Autodesk Fusion 360 part; units mm, degrees
(part 7 of 11)
  spline S10 degree 5 poles (-13.755, -25.3425) (-13.7559, -25.3451) (-13.7577, -25.3503) (-13.7602, -25.3581) (-13.7631, -25.3687) (-13.7662, -25.3821) (-13.769, -25.3956) (-13.7716, -25.4092) (-13.774, -25.4229) (-13.7763, -25.4365) (-13.7786, -25.4502) (-13.7807, -25.464) (-13.7827, -25.4778) (-13.7845, -25.4916) (-13.7861, -25.5055) (-13.7876, -25.5194) (-13.7889, -25.5334) (-13.7901, -25.5475) (-13.7912, -25.5615) (-13.7921, -25.5756) (-13.793, -25.5897) (-13.7938, -25.6039) (-13.7945, -25.618) (-13.795, -25.6322) (-13.7955, -25.6465) (-13.7958, -25.6607) (-13.796, -25.675) (-13.7962, -25.6894) (-13.7962, -25.7037) (-13.7961, -25.7181) (-13.796, -25.7325) (-13.7957, -25.7469) (-13.7954, -25.7613) (-13.7949, -25.7758) (-13.7944, -25.7903) (-13.7938, -25.8048) (-13.7931, -25.8193) (-13.7923, -25.8339) (-13.7914, -25.8484) (-13.7905, -25.863) (-13.7894, -25.8776) (-13.7883, -25.8923) (-13.7871, -25.9069) (-13.7857, -25.9216) (-13.7844, -25.9362) (-13.7829, -25.9509) (-13.7813, -25.9656) (-13.7797, -25.9804) (-13.778, -25.9951) (-13.7762, -26.0099) (-13.7743, -26.0247) (-13.7724, -26.0394) (-13.7704, -26.0542) (-13.7683, -26.0691) (-13.7661, -26.0839) (-13.7638, -26.0987) (-13.7615, -26.1136) (-13.7591, -26.1285) (-13.7566, -26.1433) (-13.754, -26.1582) (-13.7514, -26.1731) (-13.7487, -26.1881) (-13.7459, -26.203) (-13.743, -26.2179) (-13.7401, -26.2329) (-13.7371, -26.2478) (-13.734, -26.2628) (-13.7309, -26.2778) (-13.7277, -26.2928) (-13.7244, -26.3078) (-13.721, -26.3228) (-13.7183, -26.3348) (-13.7162, -26.3438) (-13.7148, -26.3498) (-13.714, -26.3528) knots 0 0 0 0 0 0 0.01428571 0.02857143 0.04285714 0.05714286 0.07142857 0.08571429 0.1 0.11428571 0.12857143 0.14285714 0.15714286 0.17142857 0.18571429 0.2 0.21428571 0.22857143 0.24285714 0.25714286 0.27142857 0.28571429 0.3 0.31428571 0.32857143 0.34285714 0.35714286 0.37142857 0.38571429 0.4 0.41428571 0.42857143 0.44285714 0.45714286 0.47142857 0.48571429 0.5 0.51428571 0.52857143 0.54285714 0.55714286 0.57142857 0.58571429 0.6 0.61428571 0.62857143 0.64285714 0.65714286 0.67142857 0.68571429 0.7 0.71428571 0.72857143 0.74285714 0.75714286 0.77142857 0.78571429 0.8 0.81428571 0.82857143 0.84285714 0.85714286 0.87142857 0.88571429 0.9 0.91428571 0.92857143 0.94285714 0.95714286 0.97142857 0.98571429 1 1 1 1 1 1
  arc A22 (-13.714, -26.3528) -> (-13.3339, -26.4547) centre (-11.6741, -19.5) ccw
  spline S11 degree 5 poles (-13.3339, -26.4547) (-13.3318, -26.4524) (-13.3276, -26.4479) (-13.3213, -26.4412) (-13.3129, -26.4321) (-13.3025, -26.4208) (-13.2921, -26.4095) (-13.2818, -26.3981) (-13.2716, -26.3867) (-13.2615, -26.3753) (-13.2514, -26.3638) (-13.2414, -26.3524) (-13.2314, -26.3408) (-13.2216, -26.3293) (-13.2118, -26.3177) (-13.202, -26.3062) (-13.1924, -26.2945) (-13.1828, -26.2829) (-13.1732, -26.2712) (-13.1638, -26.2595) (-13.1544, -26.2478) (-13.1451, -26.236) (-13.1359, -26.2243) (-13.1267, -26.2125) (-13.1176, -26.2006) (-13.1086, -26.1888) (-13.0997, -26.1769) (-13.0908, -26.165) (-13.0821, -26.153) (-13.0734, -26.1411) (-13.0648, -26.1291) (-13.0562, -26.117) (-13.0478, -26.105) (-13.0394, -26.0929) (-13.0311, -26.0808) (-13.0229, -26.0687) (-13.0147, -26.0565) (-13.0067, -26.0444) (-12.9987, -26.0322) (-12.9908, -26.0199) (-12.9831, -26.0077) (-12.9754, -25.9954) (-12.9678, -25.9831) (-12.9602, -25.9708) (-12.9528, -25.9584) (-12.9455, -25.946) (-12.9382, -25.9336) (-12.9311, -25.9211) (-12.9241, -25.9087) (-12.9171, -25.8962) (-12.9103, -25.8837) (-12.9035, -25.8711) (-12.8969, -25.8585) (-12.8904, -25.8459) (-12.884, -25.8333) (-12.8777, -25.8206) (-12.8715, -25.8079) (-12.8654, -25.7952) (-12.8594, -25.7825) (-12.8536, -25.7697) (-12.8479, -25.7569) (-12.8423, -25.7441) (-12.837, -25.7312) (-12.8318, -25.7182) (-12.8268, -25.7053) (-12.8219, -25.6923) (-12.817, -25.6793) (-12.8123, -25.6662) (-12.8077, -25.6532) (-12.8034, -25.6401) (-12.7994, -25.6269) (-12.7967, -25.6163) (-12.7949, -25.6083) (-12.7938, -25.6029) (-12.7933, -25.6002) knots -1 -1 -1 -1 -1 -1 -0.98571429 -0.97142857 -0.95714286 -0.94285714 -0.92857143 -0.91428571 -0.9 -0.88571429 -0.87142857 -0.85714286 -0.84285714 -0.82857143 -0.81428571 -0.8 -0.78571429 -0.77142857 -0.75714286 -0.74285714 -0.72857143 -0.71428571 -0.7 -0.68571429 -0.67142857 -0.65714286 -0.64285714 -0.62857143 -0.61428571 -0.6 -0.58571429 -0.57142857 -0.55714286 -0.54285714 -0.52857143 -0.51428571 -0.5 -0.48571429 -0.47142857 -0.45714286 -0.44285714 -0.42857143 -0.41428571 -0.4 -0.38571429 -0.37142857 -0.35714286 -0.34285714 -0.32857143 -0.31428571 -0.3 -0.28571429 -0.27142857 -0.25714286 -0.24285714 -0.22857143 -0.21428571 -0.2 -0.18571429 -0.17142857 -0.15714286 -0.14285714 -0.12857143 -0.11428571 -0.1 -0.08571429 -0.07142857 -0.05714286 -0.04285714 -0.02857143 -0.01428571 0 0 0 0 0 0
  line L11 (-12.7933, -25.6002) -> (-12.7808, -25.5328)
  arc A23 (-12.4999, -25.331) -> (-12.7808, -25.5328) centre (-12.535, -25.5785) ccw
  arc A24 (-12.4999, -25.331) -> (-12.3857, -25.3461) centre (-11.6741, -19.5) ccw
  arc A25 (-12.1666, -25.6137) -> (-12.3857, -25.3461) centre (-12.4159, -25.5942) ccw
  line L12 (-12.1666, -25.6137) -> (-12.172, -25.682)
  spline S12 degree 5 poles (-12.172, -25.682) (-12.1722, -25.6847) (-12.1725, -25.6902) (-12.1729, -25.6984) (-12.173, -25.7094) (-12.1725, -25.7232) (-12.1717, -25.7369) (-12.1707, -25.7507) (-12.1695, -25.7645) (-12.1682, -25.7783) (-12.1668, -25.7921) (-12.1653, -25.806) (-12.1637, -25.8198) (-12.1618, -25.8336) (-12.1598, -25.8475) (-12.1576, -25.8613) (-12.1553, -25.8752) (-12.1528, -25.889) (-12.1502, -25.9029) (-12.1475, -25.9168) (-12.1447, -25.9306) (-12.1418, -25.9445) (-12.1388, -25.9583) (-12.1356, -25.9722) (-12.1324, -25.9861) (-12.129, -25.9999) (-12.1255, -26.0138) (-12.1219, -26.0277) (-12.1182, -26.0415) (-12.1145, -26.0554) (-12.1106, -26.0693) (-12.1066, -26.0831) (-12.1025, -26.097) (-12.0984, -26.1109) (-12.0941, -26.1247) (-12.0898, -26.1386) (-12.0853, -26.1524) (-12.0808, -26.1663) (-12.0762, -26.1801) (-12.0715, -26.194) (-12.0667, -26.2078) (-12.0618, -26.2216) (-12.0568, -26.2355) (-12.0518, -26.2493) (-12.0466, -26.2631) (-12.0414, -26.2769) (-12.0361, -26.2907) (-12.0307, -26.3045) (-12.0253, -26.3183) (-12.0197, -26.3321) (-12.0141, -26.3459) (-12.0084, -26.3597) (-12.0026, -26.3735) (-11.9967, -26.3872) (-11.9908, -26.401) (-11.9847, -26.4147) (-11.9786, -26.4285) (-11.9725, -26.4422) (-11.9662, -26.456) (-11.9599, -26.4697) (-11.9535, -26.4834) (-11.947, -26.4971) (-11.9404, -26.5108) (-11.9338, -26.5245) (-11.9271, -26.5382) (-11.9203, -26.5519) (-11.9135, -26.5655) (-11.9066, -26.5792) (-11.8996, -26.5928) (-11.8925, -26.6065) (-11.8854, -26.6201) (-11.8796, -26.631) (-11.8753, -26.6391) (-11.8724, -26.6446) (-11.8709, -26.6473) knots 0 0 0 0 0 0 0.01428571 0.02857143 0.04285714 0.05714286 0.07142857 0.08571429 0.1 0.11428571 0.12857143 0.14285714 0.15714286 0.17142857 0.18571429 0.2 0.21428571 0.22857143 0.24285714 0.25714286 0.27142857 0.28571429 0.3 0.31428571 0.32857143 0.34285714 0.35714286 0.37142857 0.38571429 0.4 0.41428571 0.42857143 0.44285714 0.45714286 0.47142857 0.48571429 0.5 0.51428571 0.52857143 0.54285714 0.55714286 0.57142857 0.58571429 0.6 0.61428571 0.62857143 0.64285714 0.65714286 0.67142857 0.68571429 0.7 0.71428571 0.72857143 0.74285714 0.75714286 0.77142857 0.78571429 0.8 0.81428571 0.82857143 0.84285714 0.85714286 0.87142857 0.88571429 0.9 0.91428571 0.92857143 0.94285714 0.95714286 0.97142857 0.98571429 1 1 1 1 1 1
  arc A26 (-11.8709, -26.6473) -> (-11.4774, -26.6473) centre (-11.6741, -19.5) ccw
  spline S13 degree 5 poles (-11.4774, -26.6473) (-11.4759, -26.6446) (-11.473, -26.6391) (-11.4687, -26.631) (-11.4629, -26.6201) (-11.4558, -26.6065) (-11.4487, -26.5928) (-11.4417, -26.5792) (-11.4348, -26.5655) (-11.4279, -26.5519) (-11.4212, -26.5382) (-11.4145, -26.5245) (-11.4078, -26.5108) (-11.4013, -26.4971) (-11.3948, -26.4834) (-11.3884, -26.4697) (-11.3821, -26.456) (-11.3758, -26.4422) (-11.3696, -26.4285) (-11.3635, -26.4147) (-11.3575, -26.401) (-11.3516, -26.3872) (-11.3457, -26.3735) (-11.3399, -26.3597) (-11.3342, -26.3459) (-11.3286, -26.3321) (-11.323, -26.3183) (-11.3176, -26.3045) (-11.3122, -26.2907) (-11.3069, -26.2769) (-11.3016, -26.2631) (-11.2965, -26.2493) (-11.2915, -26.2355) (-11.2865, -26.2216) (-11.2816, -26.2078) (-11.2768, -26.194) (-11.2721, -26.1801) (-11.2675, -26.1663) (-11.2629, -26.1524) (-11.2585, -26.1386) (-11.2541, -26.1247) (-11.2499, -26.1109) (-11.2457, -26.097) (-11.2417, -26.0831) (-11.2377, -26.0693) (-11.2338, -26.0554) (-11.23, -26.0415) (-11.2264, -26.0277) (-11.2228, -26.0138) (-11.2193, -25.9999) (-11.2159, -25.9861) (-11.2127, -25.9722) (-11.2095, -25.9583) (-11.2065, -25.9445) (-11.2036, -25.9306) (-11.2008, -25.9168) (-11.1981, -25.9029) (-11.1955, -25.889) (-11.193, -25.8752) (-11.1907, -25.8613) (-11.1885, -25.8475) (-11.1864, -25.8336) (-11.1846, -25.8198) (-11.183, -25.806) (-11.1815, -25.7921) (-11.1801, -25.7783) (-11.1788, -25.7645) (-11.1776, -25.7507) (-11.1765, -25.7369) (-11.1757, -25.7232) (-11.1753, -25.7094) (-11.1754, -25.6984) (-11.1757, -25.6902) (-11.1761, -25.6847) (-11.1763, -25.682) knots -1 -1 -1 -1 -1 -1 -0.98571429 -0.97142857 -0.95714286 -0.94285714 -0.92857143 -0.91428571 -0.9 -0.88571429 -0.87142857 -0.85714286 -0.84285714 -0.82857143 -0.81428571 -0.8 -0.78571429 -0.77142857 -0.75714286 -0.74285714 -0.72857143 -0.71428571 -0.7 -0.68571429 -0.67142857 -0.65714286 -0.64285714 -0.62857143 -0.61428571 -0.6 -0.58571429 -0.57142857 -0.55714286 -0.54285714 -0.52857143 -0.51428571 -0.5 -0.48571429 -0.47142857 -0.45714286 -0.44285714 -0.42857143 -0.41428571 -0.4 -0.38571429 -0.37142857 -0.35714286 -0.34285714 -0.32857143 -0.31428571 -0.3 -0.28571429 -0.27142857 -0.25714286 -0.24285714 -0.22857143 -0.21428571 -0.2 -0.18571429 -0.17142857 -0.15714286 -0.14285714 -0.12857143 -0.11428571 -0.1 -0.08571429 -0.07142857 -0.05714286 -0.04285714 -0.02857143 -0.01428571 0 0 0 0 0 0
  line L13 (-11.1763, -25.682) -> (-11.1816, -25.6137)
  arc A27 (-10.9626, -25.3461) -> (-11.1816, -25.6137) centre (-10.9324, -25.5942) ccw
  arc A28 (-10.9626, -25.3461) -> (-10.8484, -25.331) centre (-11.6741, -19.5) ccw
  arc A29 (-10.5675, -25.5328) -> (-10.8484, -25.331) centre (-10.8133, -25.5785) ccw
  line L14 (-10.5675, -25.5328) -> (-10.555, -25.6002)
  spline S14 degree 5 poles (-10.555, -25.6002) (-10.5545, -25.6029) (-10.5534, -25.6083) (-10.5516, -25.6163) (-10.5488, -25.6269) (-10.5449, -25.6401) (-10.5405, -25.6532) (-10.536, -25.6662) (-10.5312, -25.6793) (-10.5264, -25.6923) (-10.5215, -25.7053) (-10.5165, -25.7182) (-10.5113, -25.7312) (-10.5059, -25.7441) (-10.5004, -25.7569) (-10.4947, -25.7697) (-10.4888, -25.7825) (-10.4829, -25.7952) (-10.4768, -25.8079) (-10.4706, -25.8206) (-10.4643, -25.8333) (-10.4579, -25.8459) (-10.4514, -25.8585) (-10.4448, -25.8711) (-10.438, -25.8837) (-10.4312, -25.8962) (-10.4242, -25.9087) (-10.4172, -25.9211) (-10.41, -25.9336) (-10.4028, -25.946) (-10.3955, -25.9584) (-10.388, -25.9708) (-10.3805, -25.9831) (-10.3729, -25.9954) (-10.3652, -26.0077) (-10.3574, -26.0199) (-10.3496, -26.0322) (-10.3416, -26.0444) (-10.3335, -26.0565) (-10.3254, -26.0687) (-10.3172, -26.0808) (-10.3089, -26.0929) (-10.3005, -26.105) (-10.2921, -26.117) (-10.2835, -26.1291) (-10.2749, -26.1411) (-10.2662, -26.153) (-10.2574, -26.165) (-10.2486, -26.1769) (-10.2396, -26.1888) (-10.2306, -26.2006) (-10.2216, -26.2125) (-10.2124, -26.2243) (-10.2032, -26.236) (-10.1939, -26.2478) (-10.1845, -26.2595) (-10.175, -26.2712) (-10.1655, -26.2829) (-10.1559, -26.2945) (-10.1463, -26.3062) (-10.1365, -26.3177) (-10.1267, -26.3293) (-10.1168, -26.3408) (-10.1069, -26.3524) (-10.0969, -26.3638) (-10.0868, -26.3753) (-10.0767, -26.3867) (-10.0664, -26.3981) (-10.0562, -26.4095) (-10.0458, -26.4208) (-10.0354, -26.4321) (-10.027, -26.4412) (-10.0207, -26.4479) (-10.0164, -26.4524) (-10.0143, -26.4547) knots 0 0 0 0 0 0 0.01428571 0.02857143 0.04285714 0.05714286 0.07142857 0.08571429 0.1 0.11428571 0.12857143 0.14285714 0.15714286 0.17142857 0.18571429 0.2 0.21428571 0.22857143 0.24285714 0.25714286 0.27142857 0.28571429 0.3 0.31428571 0.32857143 0.34285714 0.35714286 0.37142857 0.38571429 0.4 0.41428571 0.42857143 0.44285714 0.45714286 0.47142857 0.48571429 0.5 0.51428571 0.52857143 0.54285714 0.55714286 0.57142857 0.58571429 0.6 0.61428571 0.62857143 0.64285714 0.65714286 0.67142857 0.68571429 0.7 0.71428571 0.72857143 0.74285714 0.75714286 0.77142857 0.78571429 0.8 0.81428571 0.82857143 0.84285714 0.85714286 0.87142857 0.88571429 0.9 0.91428571 0.92857143 0.94285714 0.95714286 0.97142857 0.98571429 1 1 1 1 1 1
  arc A30 (-10.0143, -26.4547) -> (-9.6342, -26.3528) centre (-11.6741, -19.5) ccw
  spline S15 degree 5 poles (-9.6342, -26.3528) (-9.6335, -26.3498) (-9.6321, -26.3438) (-9.63, -26.3348) (-9.6273, -26.3228) (-9.6239, -26.3078) (-9.6206, -26.2928) (-9.6174, -26.2778) (-9.6142, -26.2628) (-9.6112, -26.2478) (-9.6082, -26.2329) (-9.6052, -26.2179) (-9.6024, -26.203) (-9.5996, -26.1881) (-9.5969, -26.1731) (-9.5942, -26.1582) (-9.5917, -26.1433) (-9.5892, -26.1285) (-9.5868, -26.1136) (-9.5845, -26.0987) (-9.5822, -26.0839) (-9.58, -26.0691) (-9.5779, -26.0542) (-9.5759, -26.0394) (-9.5739, -26.0247) (-9.5721, -26.0099) (-9.5703, -25.9951) (-9.5686, -25.9804) (-9.5669, -25.9656) (-9.5654, -25.9509) (-9.5639, -25.9362) (-9.5625, -25.9216) (-9.5612, -25.9069) (-9.56, -25.8923) (-9.5589, -25.8776) (-9.5578, -25.863) (-9.5569, -25.8484) (-9.556, -25.8339) (-9.5552, -25.8193) (-9.5545, -25.8048) (-9.5539, -25.7903) (-9.5533, -25.7758) (-9.5529, -25.7613) (-9.5526, -25.7469) (-9.5523, -25.7325) (-9.5522, -25.7181) (-9.5521, -25.7037) (-9.5521, -25.6894) (-9.5523, -25.675) (-9.5525, -25.6607) (-9.5528, -25.6465) (-9.5533, -25.6322) (-9.5538, -25.618) (-9.5545, -25.6039) (-9.5553, -25.5897) (-9.5561, -25.5756) (-9.5571, -25.5615) (-9.5582, -25.5475) (-9.5594, -25.5334) (-9.5607, -25.5194) (-9.5622, -25.5055) (-9.5638, -25.4916) (-9.5656, -25.4778) (-9.5676, -25.464) (-9.5697, -25.4502) (-9.572, -25.4365) (-9.5743, -25.4229) (-9.5767, -25.4092) (-9.5793, -25.3956) (-9.5821, -25.3821) (-9.5852, -25.3687) (-9.5881, -25.3581) (-9.5906, -25.3503) (-9.5924, -25.3451) (-9.5933, -25.3425) knots -1 -1 -1 -1 -1 -1 -0.98571429 -0.97142857 -0.95714286 -0.94285714 -0.92857143 -0.91428571 -0.9 -0.88571429 -0.87142857 -0.85714286 -0.84285714 -0.82857143 -0.81428571 -0.8 -0.78571429 -0.77142857 -0.75714286 -0.74285714 -0.72857143 -0.71428571 -0.7 -0.68571429 -0.67142857 -0.65714286 -0.64285714 -0.62857143 -0.61428571 -0.6 -0.58571429 -0.57142857 -0.55714286 -0.54285714 -0.52857143 -0.51428571 -0.5 -0.48571429 -0.47142857 -0.45714286 -0.44285714 -0.42857143 -0.41428571 -0.4 -0.38571429 -0.37142857 -0.35714286 -0.34285714 -0.32857143 -0.31428571 -0.3 -0.28571429 -0.27142857 -0.25714286 -0.24285714 -0.22857143 -0.21428571 -0.2 -0.18571429 -0.17142857 -0.15714286 -0.14285714 -0.12857143 -0.11428571 -0.1 -0.08571429 -0.07142857 -0.05714286 -0.04285714 -0.02857143 -0.01428571 0 0 0 0 0 0
  line L15 (-9.5933, -25.3425) -> (-9.6161, -25.2779)
  arc A31 (-9.4738, -24.9627) -> (-9.6161, -25.2779) centre (-9.3804, -25.1946) ccw
  arc A32 (-9.4738, -24.9627) -> (-9.3673, -24.9186) centre (-11.6741, -19.5) ccw
  arc A33 (-9.0438, -25.0408) -> (-9.3673, -24.9186) centre (-9.2694, -25.1486) ccw
  line L16 (-9.0438, -25.0408) -> (-9.0143, -25.1026)
  spline S16 degree 5 poles (-9.0143, -25.1026) (-9.0131, -25.1051) (-9.0107, -25.1101) (-9.0069, -25.1174) (-9.0014, -25.1269) (-8.9942, -25.1386) (-8.9866, -25.1501) (-8.9788, -25.1616) (-8.9709, -25.1729) (-8.9628, -25.1842) (-8.9547, -25.1955) (-8.9465, -25.2067) (-8.9382, -25.2179) (-8.9297, -25.2289) (-8.921, -25.2399) (-8.9122, -25.2508) (-8.9032, -25.2616) (-8.8941, -25.2724) (-8.885, -25.2831) (-8.8757, -25.2937) (-8.8663, -25.3044) (-8.8569, -25.3149) (-8.8473, -25.3254) (-8.8377, -25.3358) (-8.8279, -25.3462) (-8.8181, -25.3565) (-8.8081, -25.3668) (-8.7981, -25.377) (-8.788, -25.3872) (-8.7778, -25.3973) (-8.7675, -25.4074) (-8.7571, -25.4174) (-8.7467, -25.4274) (-8.7361, -25.4373) (-8.7255, -25.4472) (-8.7148, -25.457) (-8.704, -25.4668) (-8.6932, -25.4765) (-8.6823, -25.4862) (-8.6713, -25.4958) (-8.6602, -25.5054) (-8.649, -25.5149) (-8.6378, -25.5244) (-8.6265, -25.5339) (-8.6152, -25.5433) (-8.6038, -25.5526) (-8.5923, -25.5619) (-8.5807, -25.5712) (-8.569, -25.5804) (-8.5573, -25.5896) (-8.5456, -25.5987) (-8.5337, -25.6078) (-8.5218, -25.6168) (-8.5099, -25.6258) (-8.4978, -25.6347) (-8.4858, -25.6436) (-8.4736, -25.6525) (-8.4614, -25.6613) (-8.4491, -25.6701) (-8.4368, -25.6788) (-8.4244, -25.6875) (-8.4119, -25.6961) (-8.3994, -25.7047) (-8.3868, -25.7132) (-8.3741, -25.7217) (-8.3614, -25.7302) (-8.3487, -25.7386) (-8.3359, -25.747) (-8.323, -25.7553) (-8.31, -25.7636) (-8.2971, -25.7718) (-8.2866, -25.7783) (-8.2788, -25.7832) (-8.2735, -25.7865) (-8.2709, -25.7881) knots 0 0 0 0 0 0 0.01428571 0.02857143 0.04285714 0.05714286 0.07142857 0.08571429 0.1 0.11428571 0.12857143 0.14285714 0.15714286 0.17142857 0.18571429 0.2 0.21428571 0.22857143 0.24285714 0.25714286 0.27142857 0.28571429 0.3 0.31428571 0.32857143 0.34285714 0.35714286 0.37142857 0.38571429 0.4 0.41428571 0.42857143 0.44285714 0.45714286 0.47142857 0.48571429 0.5 0.51428571 0.52857143 0.54285714 0.55714286 0.57142857 0.58571429 0.6 0.61428571 0.62857143 0.64285714 0.65714286 0.67142857 0.68571429 0.7 0.71428571 0.72857143 0.74285714 0.75714286 0.77142857 0.78571429 0.8 0.81428571 0.82857143 0.84285714 0.85714286 0.87142857 0.88571429 0.9 0.91428571 0.92857143 0.94285714 0.95714286 0.97142857 0.98571429 1 1 1 1 1 1
  arc A34 (-8.2709, -25.7881) -> (-7.9301, -25.5914) centre (-11.6741, -19.5) ccw
  spline S17 degree 5 poles (-7.9301, -25.5914) (-7.9302, -25.5883) (-7.9304, -25.5821) (-7.9307, -25.5729) (-7.9312, -25.5605) (-7.9318, -25.5452) (-7.9325, -25.5298) (-7.9333, -25.5145) (-7.9341, -25.4992) (-7.935, -25.484) (-7.936, -25.4688) (-7.937, -25.4536) (-7.9381, -25.4384) (-7.9393, -25.4232) (-7.9405, -25.4081) (-7.9418, -25.3931) (-7.9432, -25.378) (-7.9447, -25.363) (-7.9462, -25.348) (-7.9478, -25.333) (-7.9494, -25.3181) (-7.9512, -25.3032) (-7.953, -25.2884) (-7.9548, -25.2735) (-7.9568, -25.2588) (-7.9588, -25.244) (-7.9609, -25.2293) (-7.9631, -25.2146) (-7.9653, -25.2) (-7.9676, -25.1853) (-7.97, -25.1708) (-7.9725, -25.1562) (-7.975, -25.1417) (-7.9776, -25.1273) (-7.9803, -25.1128) (-7.9831, -25.0985) (-7.9859, -25.0841) (-7.9888, -25.0698) (-7.9918, -25.0556) (-7.9949, -25.0413) (-7.9981, -25.0272) (-8.0013, -25.013) (-8.0046, -24.999) (-8.008, -24.9849) (-8.0115, -24.9709) (-8.0151, -24.957) (-8.0188, -24.9431) (-8.0225, -24.9292) (-8.0263, -24.9154) (-8.0303, -24.9017) (-8.0343, -24.888) (-8.0384, -24.8744) (-8.0426, -24.8608) (-8.0469, -24.8473) (-8.0513, -24.8338) (-8.0558, -24.8204) (-8.0604, -24.807) (-8.0651, -24.7937) (-8.0699, -24.7805) (-8.0748, -24.7673) (-8.0798, -24.7542) (-8.085, -24.7412) (-8.0903, -24.7283) (-8.0958, -24.7155) (-8.1014, -24.7028) (-8.1071, -24.6902) (-8.1129, -24.6776) (-8.1188, -24.665) (-8.1247, -24.6525) (-8.1309, -24.6402) (-8.1374, -24.6281) (-8.143, -24.6186) (-8.1474, -24.6117) (-8.1505, -24.6071) (-8.152, -24.6048) knots -1 -1 -1 -1 -1 -1 -0.98571429 -0.97142857 -0.95714286 -0.94285714 -0.92857143 -0.91428571 -0.9 -0.88571429 -0.87142857 -0.85714286 -0.84285714 -0.82857143 -0.81428571 -0.8 -0.78571429 -0.77142857 -0.75714286 -0.74285714 -0.72857143 -0.71428571 -0.7 -0.68571429 -0.67142857 -0.65714286 -0.64285714 -0.62857143 -0.61428571 -0.6 -0.58571429 -0.57142857 -0.55714286 -0.54285714 -0.52857143 -0.51428571 -0.5 -0.48571429 -0.47142857 -0.45714286 -0.44285714 -0.42857143 -0.41428571 -0.4 -0.38571429 -0.37142857 -0.35714286 -0.34285714 -0.32857143 -0.31428571 -0.3 -0.28571429 -0.27142857 -0.25714286 -0.24285714 -0.22857143 -0.21428571 -0.2 -0.18571429 -0.17142857 -0.15714286 -0.14285714 -0.12857143 -0.11428571 -0.1 -0.08571429 -0.07142857 -0.05714286 -0.04285714 -0.02857143 -0.01428571 0 0 0 0 0 0
  line L17 (-8.152, -24.6048) -> (-8.1908, -24.5484)
  arc A35 (-8.1349, -24.2071) -> (-8.1908, -24.5484) centre (-7.9847, -24.4069) ccw
  arc A36 (-8.1349, -24.2071) -> (-8.0435, -24.1369) centre (-11.6741, -19.5) ccw
  arc A37 (-7.6994, -24.1713) -> (-8.0435, -24.1369) centre (-7.8894, -24.3338) ccw
  line L18 (-7.6994, -24.1713) -> (-7.6548, -24.2233)
  spline S18 degree 5 poles (-7.6548, -24.2233) (-7.6531, -24.2254) (-7.6494, -24.2295) (-7.6439, -24.2356) (-7.6361, -24.2434) (-7.6261, -24.2529) (-7.6158, -24.262) (-7.6053, -24.271) (-7.5947, -24.2799) (-7.584, -24.2888) (-7.5733, -24.2976) (-7.5625, -24.3063) (-7.5515, -24.3149) (-7.5404, -24.3234) (-7.5292, -24.3318) (-7.5179, -24.34) (-7.5064, -24.3481) (-7.4949, -24.3562) (-7.4832, -24.3641) (-7.4715, -24.372) (-7.4597, -24.3799) (-7.4479, -24.3876) (-7.4359, -24.3953) (-7.4239, -24.4029) (-7.4118, -24.4104) (-7.3996, -24.4178) (-7.3873, -24.4251) (-7.375, -24.4324) (-7.3626, -24.4396) (-7.3501, -24.4467) (-7.3376, -24.4538) (-7.325, -24.4608) (-7.3123, -24.4677) (-7.2995, -24.4746) (-7.2867, -24.4814) (-7.2739, -24.4881) (-7.2609, -24.4947) (-7.2479, -24.5013) (-7.2349, -24.5078) (-7.2218, -24.5143) (-7.2086, -24.5207) (-7.1953, -24.527) (-7.1821, -24.5333) (-7.1687, -24.5395) (-7.1553, -24.5456) (-7.1418, -24.5517) (-7.1283, -24.5577) (-7.1148, -24.5637) (-7.1011, -24.5696) (-7.0875, -24.5754) (-7.0737, -24.5812) (-7.0599, -24.5869) (-7.0461, -24.5925) (-7.0322, -24.5981) (-7.0183, -24.6036) (-7.0043, -24.6091) (-6.9903, -24.6145) (-6.9762, -24.6198) (-6.9621, -24.6251) (-6.9479, -24.6304) (-6.9337, -24.6355) (-6.9194, -24.6406) (-6.9051, -24.6457) (-6.8907, -24.6507) (-6.8763, -24.6556) (-6.8618, -24.6605) (-6.8473, -24.6653) (-6.8328, -24.6701) (-6.8182, -24.6748) (-6.8035, -24.6794) (-6.7889, -24.684) (-6.7771, -24.6877) (-6.7682, -24.6904) (-6.7623, -24.6921) (-6.7594, -24.693) knots 0 0 0 0 0 0 0.01428571 0.02857143 0.04285714 0.05714286 0.07142857 0.08571429 0.1 0.11428571 0.12857143 0.14285714 0.15714286 0.17142857 0.18571429 0.2 0.21428571 0.22857143 0.24285714 0.25714286 0.27142857 0.28571429 0.3 0.31428571 0.32857143 0.34285714 0.35714286 0.37142857 0.38571429 0.4 0.41428571 0.42857143 0.44285714 0.45714286 0.47142857 0.48571429 0.5 0.51428571 0.52857143 0.54285714 0.55714286 0.57142857 0.58571429 0.6 0.61428571 0.62857143 0.64285714 0.65714286 0.67142857 0.68571429 0.7 0.71428571 0.72857143 0.74285714 0.75714286 0.77142857 0.78571429 0.8 0.81428571 0.82857143 0.84285714 0.85714286 0.87142857 0.88571429 0.9 0.91428571 0.92857143 0.94285714 0.95714286 0.97142857 0.98571429 1 1 1 1 1 1
  arc A38 (-6.7594, -24.693) -> (-6.4811, -24.4148) centre (-11.6741, -19.5) ccw
  spline S19 degree 5 poles (-6.4811, -24.4148) (-6.482, -24.4118) (-6.4838, -24.4059) (-6.4865, -24.3971) (-6.4901, -24.3853) (-6.4947, -24.3706) (-6.4993, -24.356) (-6.504, -24.3414) (-6.5088, -24.3268) (-6.5136, -24.3123) (-6.5185, -24.2979) (-6.5234, -24.2834) (-6.5284, -24.2691) (-6.5335, -24.2548) (-6.5386, -24.2405) (-6.5438, -24.2263) (-6.549, -24.2121) (-6.5543, -24.198) (-6.5596, -24.1839) (-6.565, -24.1698) (-6.5705, -24.1558) (-6.576, -24.1419) (-6.5816, -24.128) (-6.5873, -24.1142) (-6.593, -24.1004) (-6.5988, -24.0867) (-6.6046, -24.073) (-6.6105, -24.0594) (-6.6164, -24.0458) (-6.6224, -24.0323) (-6.6285, -24.0188) (-6.6347, -24.0054) (-6.6409, -23.9921) (-6.6471, -23.9788) (-6.6534, -23.9656) (-6.6598, -23.9524) (-6.6663, -23.9393) (-6.6728, -23.9262) (-6.6794, -23.9132) (-6.6861, -23.9003) (-6.6928, -23.8874) (-6.6996, -23.8746) (-6.7064, -23.8619) (-6.7134, -23.8492) (-6.7203, -23.8366) (-6.7274, -23.824) (-6.7345, -23.8115) (-6.7417, -23.7991) (-6.749, -23.7868) (-6.7564, -23.7745) (-6.7638, -23.7623) (-6.7713, -23.7502) (-6.7789, -23.7382) (-6.7865, -23.7263) (-6.7943, -23.7144) (-6.8021, -23.7026) (-6.81, -23.6909) (-6.818, -23.6793) (-6.826, -23.6677) (-6.8341, -23.6563) (-6.8424, -23.6449) (-6.8507, -23.6337) (-6.8592, -23.6226) (-6.8678, -23.6117) (-6.8765, -23.6008) (-6.8853, -23.5901) (-6.8942, -23.5794) (-6.9031, -23.5688) (-6.9121, -23.5583) (-6.9213, -23.548) (-6.9307, -23.538) (-6.9385, -23.5303) (-6.9446, -23.5247) (-6.9487, -23.5211) (-6.9508, -23.5193) knots -1 -1 -1 -1 -1 -1 -0.98571429 -0.97142857 -0.95714286 -0.94285714 -0.92857143 -0.91428571 -0.9 -0.88571429 -0.87142857 -0.85714286 -0.84285714 -0.82857143 -0.81428571 -0.8 -0.78571429 -0.77142857 -0.75714286 -0.74285714 -0.72857143 -0.71428571 -0.7 -0.68571429 -0.67142857 -0.65714286 -0.64285714 -0.62857143 -0.61428571 -0.6 -0.58571429 -0.57142857 -0.55714286 -0.54285714 -0.52857143 -0.51428571 -0.5 -0.48571429 -0.47142857 -0.45714286 -0.44285714 -0.42857143 -0.41428571 -0.4 -0.38571429 -0.37142857 -0.35714286 -0.34285714 -0.32857143 -0.31428571 -0.3 -0.28571429 -0.27142857 -0.25714286 -0.24285714 -0.22857143 -0.21428571 -0.2 -0.18571429 -0.17142857 -0.15714286 -0.14285714 -0.12857143 -0.11428571 -0.1 -0.08571429 -0.07142857 -0.05714286 -0.04285714 -0.02857143 -0.01428571 0 0 0 0 0 0
  line L19 (-6.9508, -23.5193) -> (-7.0029, -23.4748)
  arc A39 (-7.0372, -23.1307) -> (-7.0029, -23.4748) centre (-6.8404, -23.2848) ccw
  arc A40 (-7.0372, -23.1307) -> (-6.9671, -23.0392) centre (-11.6741, -19.5) ccw
  arc A41 (-6.6258, -22.9833) -> (-6.9671, -23.0392) centre (-6.7672, -23.1895) ccw
  line L20 (-6.6258, -22.9833) -> (-6.5693, -23.0221)
  spline S20 degree 5 poles (-6.5693, -23.0221) (-6.567, -23.0237) (-6.5625, -23.0267) (-6.5555, -23.0311) (-6.546, -23.0367) (-6.5339, -23.0432) (-6.5216, -23.0494) (-6.5091, -23.0554) (-6.4966, -23.0612) (-6.484, -23.067) (-6.4713, -23.0728) (-6.4586, -23.0784) (-6.4458, -23.0838) (-6.4329, -23.0892) (-6.4199, -23.0943) (-6.4068, -23.0994) (-6.3936, -23.1043) (-6.3804, -23.109) (-6.3671, -23.1137) (-6.3537, -23.1183) (-6.3403, -23.1228) (-6.3269, -23.1272) (-6.3134, -23.1315) (-6.2998, -23.1358) (-6.2861, -23.1399) (-6.2724, -23.1439) (-6.2587, -23.1478) (-6.2449, -23.1516) (-6.231, -23.1554) (-6.2171, -23.159) (-6.2032, -23.1626) (-6.1892, -23.1661) (-6.1752, -23.1695) (-6.1611, -23.1728) (-6.147, -23.1761) (-6.1328, -23.1792) (-6.1186, -23.1823) (-6.1043, -23.1853) (-6.09, -23.1882) (-6.0757, -23.1911) (-6.0613, -23.1938) (-6.0469, -23.1965) (-6.0324, -23.1991) (-6.0179, -23.2017) (-6.0034, -23.2041) (-5.9888, -23.2065) (-5.9742, -23.2088) (-5.9595, -23.2111) (-5.9449, -23.2132) (-5.9301, -23.2153) (-5.9154, -23.2173) (-5.9006, -23.2193) (-5.8858, -23.2212) (-5.8709, -23.223) (-5.856, -23.2247) (-5.8411, -23.2264) (-5.8261, -23.228) (-5.8112, -23.2295) (-5.7961, -23.2309) (-5.7811, -23.2323) (-5.766, -23.2336) (-5.7509, -23.2349) (-5.7358, -23.236) (-5.7206, -23.2371) (-5.7054, -23.2382) (-5.6902, -23.2391) (-5.6749, -23.24) (-5.6596, -23.2409) (-5.6443, -23.2417) (-5.629, -23.2424) (-5.6136, -23.243) (-5.6013, -23.2434) (-5.592, -23.2438) (-5.5859, -23.2439) (-5.5828, -23.244) knots 0 0 0 0 0 0 0.01428571 0.02857143 0.04285714 0.05714286 0.07142857 0.08571429 0.1 0.11428571 0.12857143 0.14285714 0.15714286 0.17142857 0.18571429 0.2 0.21428571 0.22857143 0.24285714 0.25714286 0.27142857 0.28571429 0.3 0.31428571 0.32857143 0.34285714 0.35714286 0.37142857 0.38571429 0.4 0.41428571 0.42857143 0.44285714 0.45714286 0.47142857 0.48571429 0.5 0.51428571 0.52857143 0.54285714 0.55714286 0.57142857 0.58571429 0.6 0.61428571 0.62857143 0.64285714 0.65714286 0.67142857 0.68571429 0.7 0.71428571 0.72857143 0.74285714 0.75714286 0.77142857 0.78571429 0.8 0.81428571 0.82857143 0.84285714 0.85714286 0.87142857 0.88571429 0.9 0.91428571 0.92857143 0.94285714 0.95714286 0.97142857 0.98571429 1 1 1 1 1 1
  arc A42 (-5.5828, -23.244) -> (-5.386, -22.9033) centre (-11.6741, -19.5) ccw
  spline S21 degree 5 poles (-5.386, -22.9033) (-5.3877, -22.9006) (-5.3909, -22.8954) (-5.3958, -22.8875) (-5.4023, -22.8771) (-5.4106, -22.8641) (-5.4189, -22.8512) (-5.4272, -22.8383) (-5.4355, -22.8255) (-5.444, -22.8127) (-5.4524, -22.8) (-5.4609, -22.7874) (-5.4694, -22.7748) (-5.478, -22.7623) (-5.4867, -22.7498) (-5.4953, -22.7374) (-5.5041, -22.725) (-5.5128, -22.7128) (-5.5216, -22.7005) (-5.5305, -22.6884) (-5.5394, -22.6763) (-5.5483, -22.6643) (-5.5573, -22.6523) (-5.5664, -22.6404) (-5.5754, -22.6286) (-5.5846, -22.6168) (-5.5937, -22.6051) (-5.603, -22.5935) (-5.6122, -22.5819) (-5.6215, -22.5704) (-5.6309, -22.559) (-5.6403, -22.5476) (-5.6497, -22.5363) (-5.6592, -22.5251) (-5.6688, -22.5139) (-5.6783, -22.5029) (-5.688, -22.4919) (-5.6977, -22.481) (-5.7074, -22.4701) (-5.7172, -22.4593) (-5.727, -22.4486) (-5.7368, -22.438) (-5.7468, -22.4275) (-5.7567, -22.417) (-5.7668, -22.4067) (-5.7768, -22.3964) (-5.7869, -22.3862) (-5.7971, -22.376) (-5.8073, -22.366) (-5.8176, -22.3561) (-5.8279, -22.3462) (-5.8383, -22.3365) (-5.8487, -22.3268) (-5.8592, -22.3173) (-5.8698, -22.3078) (-5.8804, -22.2984) (-5.891, -22.2892) (-5.9018, -22.28) (-5.9125, -22.2709) (-5.9233, -22.262) (-5.9342, -22.2531) (-5.9452, -22.2445) (-5.9563, -22.236) (-5.9674, -22.2276) (-5.9786, -22.2194) (-5.9899, -22.2113) (-6.0012, -22.2033) (-6.0126, -22.1953) (-6.024, -22.1875) (-6.0355, -22.18) (-6.0472, -22.1727) (-6.0568, -22.1673) (-6.0641, -22.1635) (-6.069, -22.161) (-6.0715, -22.1599) knots -1 -1 -1 -1 -1 -1 -0.98571429 -0.97142857 -0.95714286 -0.94285714 -0.92857143 -0.91428571 -0.9 -0.88571429 -0.87142857 -0.85714286 -0.84285714 -0.82857143 -0.81428571 -0.8 -0.78571429 -0.77142857 -0.75714286 -0.74285714 -0.72857143 -0.71428571 -0.7 -0.68571429 -0.67142857 -0.65714286 -0.64285714 -0.62857143 -0.61428571 -0.6 -0.58571429 -0.57142857 -0.55714286 -0.54285714 -0.52857143 -0.51428571 -0.5 -0.48571429 -0.47142857 -0.45714286 -0.44285714 -0.42857143 -0.41428571 -0.4 -0.38571429 -0.37142857 -0.35714286 -0.34285714 -0.32857143 -0.31428571 -0.3 -0.28571429 -0.27142857 -0.25714286 -0.24285714 -0.22857143 -0.21428571 -0.2 -0.18571429 -0.17142857 -0.15714286 -0.14285714 -0.12857143 -0.11428571 -0.1 -0.08571429 -0.07142857 -0.05714286 -0.04285714 -0.02857143 -0.01428571 0 0 0 0 0 0
  line L21 (-6.0715, -22.1599) -> (-6.1333, -22.1303)
  arc A43 (-6.2555, -21.8068) -> (-6.1333, -22.1303) centre (-6.0255, -21.9048) ccw
  arc A44 (-6.2555, -21.8068) -> (-6.2114, -21.7004) centre (-11.6741, -19.5) ccw
  arc A45 (-5.8962, -21.558) -> (-6.2114, -21.7004) centre (-5.9795, -21.7938) ccw
  line L22 (-5.8962, -21.558) -> (-5.8317, -21.5809)
  spline S22 degree 5 poles (-5.8317, -21.5809) (-5.8291, -21.5818) (-5.8239, -21.5835) (-5.816, -21.586) (-5.8054, -21.5889) (-5.792, -21.5921) (-5.7785, -21.5949) (-5.7649, -21.5974) (-5.7513, -21.5998) (-5.7376, -21.6022) (-5.7239, -21.6044) (-5.7102, -21.6066) (-5.6964, -21.6085) (-5.6825, -21.6103) (-5.6686, -21.612) (-5.6547, -21.6134) (-5.6407, -21.6147) (-5.6267, -21.6159) (-5.6126, -21.617) (-5.5985, -21.618) (-5.5844, -21.6189) (-5.5703, -21.6197) (-5.5561, -21.6203) (-5.5419, -21.6209) (-5.5277, -21.6213) (-5.5134, -21.6217) (-5.4991, -21.6219) (-5.4848, -21.622) (-5.4704, -21.622) (-5.4561, -21.622) (-5.4417, -21.6218) (-5.4272, -21.6216) (-5.4128, -21.6212) (-5.3983, -21.6208) (-5.3839, -21.6203) (-5.3694, -21.6197) (-5.3548, -21.619) (-5.3403, -21.6182) (-5.3257, -21.6173) (-5.3111, -21.6163) (-5.2965, -21.6153) (-5.2819, -21.6141) (-5.2672, -21.6129) (-5.2526, -21.6116) (-5.2379, -21.6102) (-5.2232, -21.6088) (-5.2085, -21.6072) (-5.1938, -21.6056) (-5.179, -21.6039) (-5.1643, -21.6021) (-5.1495, -21.6002) (-5.1347, -21.5983) (-5.1199, -21.5962) (-5.1051, -21.5941) (-5.0902, -21.5919) (-5.0754, -21.5897) (-5.0605, -21.5874) (-5.0457, -21.5849) (-5.0308, -21.5825) (-5.0159, -21.5799) (-5.001, -21.5773) (-4.9861, -21.5745) (-4.9711, -21.5718) (-4.9562, -21.5689) (-4.9413, -21.566) (-4.9263, -21.563) (-4.9113, -21.5599) (-4.8963, -21.5567) (-4.8814, -21.5535) (-4.8664, -21.5502) (-4.8514, -21.5469) (-4.8393, -21.5441) (-4.8303, -21.542) (-4.8243, -21.5406) (-4.8213, -21.5399) knots 0 0 0 0 0 0 0.01428571 0.02857143 0.04285714 0.05714286 0.07142857 0.08571429 0.1 0.11428571 0.12857143 0.14285714 0.15714286 0.17142857 0.18571429 0.2 0.21428571 0.22857143 0.24285714 0.25714286 0.27142857 0.28571429 0.3 0.31428571 0.32857143 0.34285714 0.35714286 0.37142857 0.38571429 0.4 0.41428571 0.42857143 0.44285714 0.45714286 0.47142857 0.48571429 0.5 0.51428571 0.52857143 0.54285714 0.55714286 0.57142857 0.58571429 0.6 0.61428571 0.62857143 0.64285714 0.65714286 0.67142857 0.68571429 0.7 0.71428571 0.72857143 0.74285714 0.75714286 0.77142857 0.78571429 0.8 0.81428571 0.82857143 0.84285714 0.85714286 0.87142857 0.88571429 0.9 0.91428571 0.92857143 0.94285714 0.95714286 0.97142857 0.98571429 1 1 1 1 1 1
  arc A46 (-4.8213, -21.5399) -> (-4.7195, -21.1598) centre (-11.6741, -19.5) ccw
  spline S23 degree 5 poles (-4.7195, -21.1598) (-4.7217, -21.1577) (-4.7262, -21.1535) (-4.733, -21.1471) (-4.742, -21.1388) (-4.7533, -21.1283) (-4.7647, -21.118) (-4.776, -21.1077) (-4.7874, -21.0975) (-4.7988, -21.0873) (-4.8103, -21.0773) (-4.8218, -21.0672) (-4.8333, -21.0573) (-4.8448, -21.0474) (-4.8564, -21.0376) (-4.868, -21.0279) (-4.8796, -21.0182) (-4.8912, -21.0086) (-4.9029, -20.9991) (-4.9146, -20.9896) (-4.9263, -20.9803) (-4.9381, -20.971) (-4.9499, -20.9617) (-4.9617, -20.9526) (-4.9735, -20.9435) (-4.9854, -20.9345) (-4.9973, -20.9256) (-5.0092, -20.9167) (-5.0211, -20.9079) (-5.0331, -20.8992) (-5.0451, -20.8906) (-5.0571, -20.8821) (-5.0691, -20.8736) (-5.0812, -20.8652) (-5.0933, -20.8569) (-5.1054, -20.8487) (-5.1176, -20.8406) (-5.1298, -20.8325) (-5.142, -20.8246) (-5.1542, -20.8167) (-5.1665, -20.8089) (-5.1787, -20.8012) (-5.191, -20.7936) (-5.2034, -20.7861) (-5.2157, -20.7787) (-5.2281, -20.7713) (-5.2405, -20.7641) (-5.253, -20.757) (-5.2655, -20.7499) (-5.278, -20.743) (-5.2905, -20.7361) (-5.303, -20.7294) (-5.3156, -20.7228) (-5.3282, -20.7162) (-5.3409, -20.7099) (-5.3535, -20.7036) (-5.3662, -20.6974) (-5.3789, -20.6913) (-5.3917, -20.6853) (-5.4044, -20.6794) (-5.4172, -20.6737) (-5.4301, -20.6682) (-5.443, -20.6628) (-5.4559, -20.6577) (-5.4689, -20.6526) (-5.4819, -20.6477) (-5.4949, -20.6429) (-5.5079, -20.6382) (-5.5209, -20.6336) (-5.534, -20.6293) (-5.5472, -20.6253) (-5.5578, -20.6225) (-5.5659, -20.6207) (-5.5713, -20.6197) (-5.574, -20.6192) knots -1 -1 -1 -1 -1 -1 -0.98571429 -0.97142857 -0.95714286 -0.94285714 -0.92857143 -0.91428571 -0.9 -0.88571429 -0.87142857 -0.85714286 -0.84285714 -0.82857143 -0.81428571 -0.8 -0.78571429 -0.77142857 -0.75714286 -0.74285714 -0.72857143 -0.71428571 -0.7 -0.68571429 -0.67142857 -0.65714286 -0.64285714 -0.62857143 -0.61428571 -0.6 -0.58571429 -0.57142857 -0.55714286 -0.54285714 -0.52857143 -0.51428571 -0.5 -0.48571429 -0.47142857 -0.45714286 -0.44285714 -0.42857143 -0.41428571 -0.4 -0.38571429 -0.37142857 -0.35714286 -0.34285714 -0.32857143 -0.31428571 -0.3 -0.28571429 -0.27142857 -0.25714286 -0.24285714 -0.22857143 -0.21428571 -0.2 -0.18571429 -0.17142857 -0.15714286 -0.14285714 -0.12857143 -0.11428571 -0.1 -0.08571429 -0.07142857 -0.05714286 -0.04285714 -0.02857143 -0.01428571 0 0 0 0 0 0
  line L23 (-5.574, -20.6192) -> (-5.6413, -20.6066)
  arc A47 (-5.8431, -20.3258) -> (-5.6413, -20.6066) centre (-5.5956, -20.3608) ccw
  arc A48 (-5.8431, -20.3258) -> (-5.8281, -20.2115) centre (-11.6741, -19.5) ccw
  arc A49 (-5.5605, -19.9925) -> (-5.8281, -20.2115) centre (-5.5799, -20.2417) ccw
  line L24 (-5.5605, -19.9925) -> (-5.4922, -19.9978)
  spline S24 degree 5 poles (-5.4922, -19.9978) (-5.4894, -19.998) (-5.484, -19.9984) (-5.4757, -19.9987) (-5.4647, -19.9988) (-5.451, -19.9984) (-5.4372, -19.9976) (-5.4234, -19.9965) (-5.4096, -19.9954) (-5.3958, -19.9941) (-5.382, -19.9927) (-5.3682, -19.9912) (-5.3543, -19.9895) (-5.3405, -19.9877) (-5.3267, -19.9857) (-5.3128, -19.9835) (-5.299, -19.9811) (-5.2851, -19.9786) (-5.2712, -19.976) (-5.2574, -19.9733) (-5.2435, -19.9705) (-5.2297, -19.9676) (-5.2158, -19.9646) (-5.2019, -19.9615) (-5.1881, -19.9582) (-5.1742, -19.9548) (-5.1603, -19.9514) (-5.1465, -19.9478) (-5.1326, -19.9441) (-5.1187, -19.9403) (-5.1049, -19.9364) (-5.091, -19.9325) (-5.0771, -19.9284) (-5.0633, -19.9242) (-5.0494, -19.92) (-5.0356, -19.9156) (-5.0217, -19.9112) (-5.0079, -19.9067) (-4.994, -19.902) (-4.9802, -19.8973) (-4.9663, -19.8925) (-4.9525, -19.8877) (-4.9387, -19.8827) (-4.9249, -19.8776) (-4.911, -19.8725) (-4.8972, -19.8673) (-4.8834, -19.862) (-4.8696, -19.8566) (-4.8558, -19.8511) (-4.842, -19.8456) (-4.8282, -19.8399) (-4.8145, -19.8342) (-4.8007, -19.8284) (-4.7869, -19.8226) (-4.7731, -19.8166) (-4.7594, -19.8106) (-4.7456, -19.8045) (-4.7319, -19.7983) (-4.7182, -19.7921) (-4.7045, -19.7857) (-4.6907, -19.7793) (-4.677, -19.7729) (-4.6633, -19.7663) (-4.6496, -19.7597) (-4.636, -19.753) (-4.6223, -19.7462) (-4.6086, -19.7394) (-4.595, -19.7324) (-4.5813, -19.7254) (-4.5677, -19.7184) (-4.5541, -19.7113) (-4.5432, -19.7055) (-4.535, -19.7011) (-4.5296, -19.6982) (-4.5268, -19.6968) knots 0 0 0 0 0 0 0.01428571 0.02857143 0.04285714 0.05714286 0.07142857 0.08571429 0.1 0.11428571 0.12857143 0.14285714 0.15714286 0.17142857 0.18571429 0.2 0.21428571 0.22857143 0.24285714 0.25714286 0.27142857 0.28571429 0.3 0.31428571 0.32857143 0.34285714 0.35714286 0.37142857 0.38571429 0.4 0.41428571 0.42857143 0.44285714 0.45714286 0.47142857 0.48571429 0.5 0.51428571 0.52857143 0.54285714 0.55714286 0.57142857 0.58571429 0.6 0.61428571 0.62857143 0.64285714 0.65714286 0.67142857 0.68571429 0.7 0.71428571 0.72857143 0.74285714 0.75714286 0.77142857 0.78571429 0.8 0.81428571 0.82857143 0.84285714 0.85714286 0.87142857 0.88571429 0.9 0.91428571 0.92857143 0.94285714 0.95714286 0.97142857 0.98571429 1 1 1 1 1 1
  arc A50 (-4.5268, -19.6968) -> (-4.5268, -19.3032) centre (-11.6741, -19.5) ccw
  spline S25 degree 5 poles (-4.5268, -19.3032) (-4.5296, -19.3018) (-4.535, -19.2989) (-4.5432, -19.2945) (-4.5541, -19.2887) (-4.5677, -19.2816) (-4.5813, -19.2746) (-4.595, -19.2676) (-4.6086, -19.2606) (-4.6223, -19.2538) (-4.636, -19.247) (-4.6496, -19.2403) (-4.6633, -19.2337) (-4.677, -19.2271) (-4.6907, -19.2207) (-4.7045, -19.2143) (-4.7182, -19.2079) (-4.7319, -19.2017) (-4.7456, -19.1955) (-4.7594, -19.1894) (-4.7731, -19.1834) (-4.7869, -19.1774) (-4.8007, -19.1716) (-4.8145, -19.1658) (-4.8282, -19.1601) (-4.842, -19.1544) (-4.8558, -19.1489) (-4.8696, -19.1434) (-4.8834, -19.138) (-4.8972, -19.1327) (-4.911, -19.1275) (-4.9249, -19.1224) (-4.9387, -19.1173) (-4.9525, -19.1123) (-4.9663, -19.1075) (-4.9802, -19.1027) (-4.994, -19.098) (-5.0079, -19.0933) (-5.0217, -19.0888) (-5.0356, -19.0844) (-5.0494, -19.08) (-5.0633, -19.0758) (-5.0771, -19.0716) (-5.091, -19.0675) (-5.1049, -19.0636) (-5.1187, -19.0597) (-5.1326, -19.0559) (-5.1465, -19.0522) (-5.1603, -19.0486) (-5.1742, -19.0452) (-5.1881, -19.0418) (-5.2019, -19.0385) (-5.2158, -19.0354) (-5.2297, -19.0324) (-5.2435, -19.0295) (-5.2574, -19.0267) (-5.2712, -19.024) (-5.2851, -19.0214) (-5.299, -19.0189) (-5.3128, -19.0165) (-5.3267, -19.0143) (-5.3405, -19.0123) (-5.3543, -19.0105) (-5.3682, -19.0088) (-5.382, -19.0073) (-5.3958, -19.0059) (-5.4096, -19.0046) (-5.4234, -19.0035) (-5.4372, -19.0024) (-5.451, -19.0016) (-5.4647, -19.0012) (-5.4757, -19.0013) (-5.484, -19.0016) (-5.4894, -19.002) (-5.4922, -19.0022) knots -1 -1 -1 -1 -1 -1 -0.98571429 -0.97142857 -0.95714286 -0.94285714 -0.92857143 -0.91428571 -0.9 -0.88571429 -0.87142857 -0.85714286 -0.84285714 -0.82857143 -0.81428571 -0.8 -0.78571429 -0.77142857 -0.75714286 -0.74285714 -0.72857143 -0.71428571 -0.7 -0.68571429 -0.67142857 -0.65714286 -0.64285714 -0.62857143 -0.61428571 -0.6 -0.58571429 -0.57142857 -0.55714286 -0.54285714 -0.52857143 -0.51428571 -0.5 -0.48571429 -0.47142857 -0.45714286 -0.44285714 -0.42857143 -0.41428571 -0.4 -0.38571429 -0.37142857 -0.35714286 -0.34285714 -0.32857143 -0.31428571 -0.3 -0.28571429 -0.27142857 -0.25714286 -0.24285714 -0.22857143 -0.21428571 -0.2 -0.18571429 -0.17142857 -0.15714286 -0.14285714 -0.12857143 -0.11428571 -0.1 -0.08571429 -0.07142857 -0.05714286 -0.04285714 -0.02857143 -0.01428571 0 0 0 0 0 0
  line L25 (-5.4922, -19.0022) -> (-5.5605, -19.0075)
  arc A51 (-5.8281, -18.7885) -> (-5.5605, -19.0075) centre (-5.5799, -18.7583) ccw
  arc A52 (-5.8281, -18.7885) -> (-5.8431, -18.6742) centre (-11.6741, -19.5) ccw
  arc A53 (-5.6413, -18.3934) -> (-5.8431, -18.6742) centre (-5.5956, -18.6392) ccw
  line L26 (-5.6413, -18.3934) -> (-5.574, -18.3808)
  spline S26 degree 5 poles (-5.574, -18.3808) (-5.5713, -18.3803) (-5.5659, -18.3793) (-5.5578, -18.3775) (-5.5472, -18.3747) (-5.534, -18.3707) (-5.5209, -18.3664) (-5.5079, -18.3618) (-5.4949, -18.3571) (-5.4819, -18.3523) (-5.4689, -18.3474) (-5.4559, -18.3423) (-5.443, -18.3372) (-5.4301, -18.3318) (-5.4172, -18.3263) (-5.4044, -18.3206) (-5.3917, -18.3147) (-5.3789, -18.3087) (-5.3662, -18.3026) (-5.3535, -18.2964) (-5.3409, -18.2901) (-5.3282, -18.2838) (-5.3156, -18.2772) (-5.303, -18.2706) (-5.2905, -18.2639) (-5.278, -18.257) (-5.2655, -18.2501) (-5.253, -18.243) (-5.2405, -18.2359) (-5.2281, -18.2287) (-5.2157, -18.2213) (-5.2034, -18.2139) (-5.191, -18.2064) (-5.1787, -18.1988) (-5.1665, -18.1911) (-5.1542, -18.1833) (-5.142, -18.1754) (-5.1298, -18.1675) (-5.1176, -18.1594) (-5.1054, -18.1513) (-5.0933, -18.1431) (-5.0812, -18.1348) (-5.0691, -18.1264) (-5.0571, -18.1179) (-5.0451, -18.1094) (-5.0331, -18.1008) (-5.0211, -18.0921) (-5.0092, -18.0833) (-4.9973, -18.0744) (-4.9854, -18.0655) (-4.9735, -18.0565) (-4.9617, -18.0474) (-4.9499, -18.0383) (-4.9381, -18.029) (-4.9263, -18.0197) (-4.9146, -18.0104) (-4.9029, -18.0009) (-4.8912, -17.9914) (-4.8796, -17.9818) (-4.868, -17.9721) (-4.8564, -17.9624) (-4.8448, -17.9526) (-4.8333, -17.9427) (-4.8218, -17.9328) (-4.8103, -17.9227) (-4.7988, -17.9127) (-4.7874, -17.9025) (-4.776, -17.8923) (-4.7647, -17.882) (-4.7533, -17.8717) (-4.742, -17.8612) (-4.733, -17.8529) (-4.7262, -17.8465) (-4.7217, -17.8423) (-4.7195, -17.8402) knots 0 0 0 0 0 0 0.01428571 0.02857143 0.04285714 0.05714286 0.07142857 0.08571429 0.1 0.11428571 0.12857143 0.14285714 0.15714286 0.17142857 0.18571429 0.2 0.21428571 0.22857143 0.24285714 0.25714286 0.27142857 0.28571429 0.3 0.31428571 0.32857143 0.34285714 0.35714286 0.37142857 0.38571429 0.4 0.41428571 0.42857143 0.44285714 0.45714286 0.47142857 0.48571429 0.5 0.51428571 0.52857143 0.54285714 0.55714286 0.57142857 0.58571429 0.6 0.61428571 0.62857143 0.64285714 0.65714286 0.67142857 0.68571429 0.7 0.71428571 0.72857143 0.74285714 0.75714286 0.77142857 0.78571429 0.8 0.81428571 0.82857143 0.84285714 0.85714286 0.87142857 0.88571429 0.9 0.91428571 0.92857143 0.94285714 0.95714286 0.97142857 0.98571429 1 1 1 1 1 1
  arc A54 (-4.7195, -17.8402) -> (-4.8213, -17.4601) centre (-11.6741, -19.5) ccw
  spline S27 degree 5 poles (-4.8213, -17.4601) (-4.8243, -17.4594) (-4.8303, -17.458) (-4.8393, -17.4559) (-4.8514, -17.4531) (-4.8664, -17.4498) (-4.8814, -17.4465) (-4.8963, -17.4433) (-4.9113, -17.4401) (-4.9263, -17.437) (-4.9413, -17.434) (-4.9562, -17.4311) (-4.9711, -17.4282) (-4.9861, -17.4255) (-5.001, -17.4227) (-5.0159, -17.4201) (-5.0308, -17.4175) (-5.0457, -17.4151) (-5.0605, -17.4126) (-5.0754, -17.4103) (-5.0902, -17.4081) (-5.1051, -17.4059) (-5.1199, -17.4038) (-5.1347, -17.4017) (-5.1495, -17.3998) (-5.1643, -17.3979) (-5.179, -17.3961) (-5.1938, -17.3944) (-5.2085, -17.3928) (-5.2232, -17.3912) (-5.2379, -17.3898) (-5.2526, -17.3884) (-5.2672, -17.3871) (-5.2819, -17.3859) (-5.2965, -17.3847) (-5.3111, -17.3837) (-5.3257, -17.3827) (-5.3403, -17.3818) (-5.3548, -17.381) (-5.3694, -17.3803) (-5.3839, -17.3797) (-5.3983, -17.3792) (-5.4128, -17.3788) (-5.4272, -17.3784) (-5.4417, -17.3782) (-5.4561, -17.378) (-5.4704, -17.378) (-5.4848, -17.378) (-5.4991, -17.3781) (-5.5134, -17.3783) (-5.5277, -17.3787) (-5.5419, -17.3791) (-5.5561, -17.3797) (-5.5703, -17.3803) (-5.5844, -17.3811) (-5.5985, -17.382) (-5.6126, -17.383) (-5.6267, -17.3841) (-5.6407, -17.3853) (-5.6547, -17.3866) (-5.6686, -17.388) (-5.6825, -17.3897) (-5.6964, -17.3915) (-5.7102, -17.3934) (-5.7239, -17.3956) (-5.7376, -17.3978) (-5.7513, -17.4002) (-5.7649, -17.4026) (-5.7785, -17.4051) (-5.792, -17.4079) (-5.8054, -17.4111) (-5.816, -17.414) (-5.8239, -17.4165) (-5.8291, -17.4182) (-5.8317, -17.4191) knots -1 -1 -1 -1 -1 -1 -0.98571429 -0.97142857 -0.95714286 -0.94285714 -0.92857143 -0.91428571 -0.9 -0.88571429 -0.87142857 -0.85714286 -0.84285714 -0.82857143 -0.81428571 -0.8 -0.78571429 -0.77142857 -0.75714286 -0.74285714 -0.72857143 -0.71428571 -0.7 -0.68571429 -0.67142857 -0.65714286 -0.64285714 -0.62857143 -0.61428571 -0.6 -0.58571429 -0.57142857 -0.55714286 -0.54285714 -0.52857143 -0.51428571 -0.5 -0.48571429 -0.47142857 -0.45714286 -0.44285714 -0.42857143 -0.41428571 -0.4 -0.38571429 -0.37142857 -0.35714286 -0.34285714 -0.32857143 -0.31428571 -0.3 -0.28571429 -0.27142857 -0.25714286 -0.24285714 -0.22857143 -0.21428571 -0.2 -0.18571429 -0.17142857 -0.15714286 -0.14285714 -0.12857143 -0.11428571 -0.1 -0.08571429 -0.07142857 -0.05714286 -0.04285714 -0.02857143 -0.01428571 0 0 0 0 0 0
  line L27 (-5.8317, -17.4191) -> (-5.8962, -17.442)
  arc A55 (-6.2114, -17.2996) -> (-5.8962, -17.442) centre (-5.9795, -17.2062) ccw
  arc A56 (-6.2114, -17.2996) -> (-6.2555, -17.1932) centre (-11.6741, -19.5) ccw
  arc A57 (-6.1333, -16.8697) -> (-6.2555, -17.1932) centre (-6.0255, -17.0952) ccw
  line L28 (-6.1333, -16.8697) -> (-6.0715, -16.8401)
  spline S28 degree 5 poles (-6.0715, -16.8401) (-6.069, -16.839) (-6.0641, -16.8365) (-6.0568, -16.8327) (-6.0472, -16.8273) (-6.0355, -16.82) (-6.024, -16.8125) (-6.0126, -16.8047) (-6.0012, -16.7967) (-5.9899, -16.7887) (-5.9786, -16.7806) (-5.9674, -16.7724) (-5.9563, -16.764) (-5.9452, -16.7555) (-5.9342, -16.7469) (-5.9233, -16.738) (-5.9125, -16.7291) (-5.9018, -16.72) (-5.891, -16.7108) (-5.8804, -16.7016) (-5.8698, -16.6922) (-5.8592, -16.6827) (-5.8487, -16.6732) (-5.8383, -16.6635) (-5.8279, -16.6538) (-5.8176, -16.6439) (-5.8073, -16.634) (-5.7971, -16.624) (-5.7869, -16.6138) (-5.7768, -16.6036) (-5.7668, -16.5933) (-5.7567, -16.583) (-5.7468, -16.5725) (-5.7368, -16.562) (-5.727, -16.5514) (-5.7172, -16.5407) (-5.7074, -16.5299) (-5.6977, -16.5191) (-5.688, -16.5081) (-5.6783, -16.4971) (-5.6688, -16.4861) (-5.6592, -16.4749) (-5.6497, -16.4637) (-5.6403, -16.4524) (-5.6309, -16.441) (-5.6215, -16.4296) (-5.6122, -16.4181) (-5.603, -16.4065) (-5.5937, -16.3949) (-5.5846, -16.3832) (-5.5754, -16.3714) (-5.5664, -16.3596) (-5.5573, -16.3477) (-5.5483, -16.3357) (-5.5394, -16.3237) (-5.5305, -16.3116) (-5.5216, -16.2995) (-5.5128, -16.2872) (-5.5041, -16.275) (-5.4953, -16.2626) (-5.4867, -16.2502) (-5.478, -16.2378) (-5.4694, -16.2252) (-5.4609, -16.2126) (-5.4524, -16.2) (-5.444, -16.1873) (-5.4355, -16.1745) (-5.4272, -16.1617) (-5.4189, -16.1488) (-5.4106, -16.1359) (-5.4023, -16.1229) (-5.3958, -16.1125) (-5.3909, -16.1046) (-5.3877, -16.0994) (-5.386, -16.0967) knots 0 0 0 0 0 0 0.01428571 0.02857143 0.04285714 0.05714286 0.07142857 0.08571429 0.1 0.11428571 0.12857143 0.14285714 0.15714286 0.17142857 0.18571429 0.2 0.21428571 0.22857143 0.24285714 0.25714286 0.27142857 0.28571429 0.3 0.31428571 0.32857143 0.34285714 0.35714286 0.37142857 0.38571429 0.4 0.41428571 0.42857143 0.44285714 0.45714286 0.47142857 0.48571429 0.5 0.51428571 0.52857143 0.54285714 0.55714286 0.57142857 0.58571429 0.6 0.61428571 0.62857143 0.64285714 0.65714286 0.67142857 0.68571429 0.7 0.71428571 0.72857143 0.74285714 0.75714286 0.77142857 0.78571429 0.8 0.81428571 0.82857143 0.84285714 0.85714286 0.87142857 0.88571429 0.9 0.91428571 0.92857143 0.94285714 0.95714286 0.97142857 0.98571429 1 1 1 1 1 1
  arc A58 (-5.386, -16.0967) -> (-5.5828, -15.756) centre (-11.6741, -19.5) ccw
  spline S29 degree 5 poles (-5.5828, -15.756) (-5.5859, -15.7561) (-5.592, -15.7562) (-5.6013, -15.7566) (-5.6136, -15.757) (-5.629, -15.7576) (-5.6443, -15.7583) (-5.6596, -15.7591) (-5.6749, -15.76) (-5.6902, -15.7609) (-5.7054, -15.7618) (-5.7206, -15.7629) (-5.7358, -15.764) (-5.7509, -15.7651) (-5.766, -15.7664) (-5.7811, -15.7677) (-5.7961, -15.7691) (-5.8112, -15.7705) (-5.8261, -15.772) (-5.8411, -15.7736) (-5.856, -15.7753) (-5.8709, -15.777) (-5.8858, -15.7788) (-5.9006, -15.7807) (-5.9154, -15.7827) (-5.9301, -15.7847) (-5.9449, -15.7868) (-5.9595, -15.7889) (-5.9742, -15.7912) (-5.9888, -15.7935) (-6.0034, -15.7959) (-6.0179, -15.7983) (-6.0324, -15.8009) (-6.0469, -15.8035) (-6.0613, -15.8062) (-6.0757, -15.8089) (-6.09, -15.8118) (-6.1043, -15.8147) (-6.1186, -15.8177) (-6.1328, -15.8208) (-6.147, -15.8239) (-6.1611, -15.8272) (-6.1752, -15.8305) (-6.1892, -15.8339) (-6.2032, -15.8374) (-6.2171, -15.841) (-6.231, -15.8446) (-6.2449, -15.8484) (-6.2587, -15.8522) (-6.2724, -15.8561) (-6.2861, -15.8601) (-6.2998, -15.8642) (-6.3134, -15.8685) (-6.3269, -15.8728) (-6.3403, -15.8772) (-6.3537, -15.8817) (-6.3671, -15.8863) (-6.3804, -15.891) (-6.3936, -15.8957) (-6.4068, -15.9006) (-6.4199, -15.9057) (-6.4329, -15.9108) (-6.4458, -15.9162) (-6.4586, -15.9216) (-6.4713, -15.9272) (-6.484, -15.933) (-6.4966, -15.9388) (-6.5091, -15.9446) (-6.5216, -15.9506) (-6.5339, -15.9568) (-6.546, -15.9633) (-6.5555, -15.9689) (-6.5625, -15.9733) (-6.567, -15.9763) (-6.5693, -15.9779) knots -1 -1 -1 -1 -1 -1 -0.98571429 -0.97142857 -0.95714286 -0.94285714 -0.92857143 -0.91428571 -0.9 -0.88571429 -0.87142857 -0.85714286 -0.84285714 -0.82857143 -0.81428571 -0.8 -0.78571429 -0.77142857 -0.75714286 -0.74285714 -0.72857143 -0.71428571 -0.7 -0.68571429 -0.67142857 -0.65714286 -0.64285714 -0.62857143 -0.61428571 -0.6 -0.58571429 -0.57142857 -0.55714286 -0.54285714 -0.52857143 -0.51428571 -0.5 -0.48571429 -0.47142857 -0.45714286 -0.44285714 -0.42857143 -0.41428571 -0.4 -0.38571429 -0.37142857 -0.35714286 -0.34285714 -0.32857143 -0.31428571 -0.3 -0.28571429 -0.27142857 -0.25714286 -0.24285714 -0.22857143 -0.21428571 -0.2 -0.18571429 -0.17142857 -0.15714286 -0.14285714 -0.12857143 -0.11428571 -0.1 -0.08571429 -0.07142857 -0.05714286 -0.04285714 -0.02857143 -0.01428571 0 0 0 0 0 0